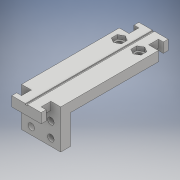
# Autodesk Inventor part: Attachment
Saved by Autodesk Inventor 2018 (Build 220112000, 112)
## iProperties
Created: 2018-05-09
Part Number: Attachment
Material: Generic
Document SubType Name: Modeling
Designer: s4321966
Density: 1 g/cm^3
Appearance: Default
Mass: 6.80777 g
Surface Area: 44.3396 cm^2
Volume: 6.80777 cm^3
Author: s4321966
Autodesk Inventor part; units mm, degrees
ref_plane "YZ Plane" through (0, 0, 0) normal (1, 0, 0) x (0, 1, 0)
ref_plane "XZ Plane" through (0, 0, 0) normal (0, 1, 0) x (-1, 0, 0)
ref_plane "XY Plane" through (0, 0, 0) normal (0, 0, 1) x (1, 0, 0)
sketch "Sketch1" plane through (0, 0, 0) normal (0, 0, 1) x (1, 0, 0)
  line L0 (0, 0) -> (20, 0)
  line L1 (20, 0) -> (20, -2.7984)
  line L2 (0, -2.7984) -> (0, 0)
  line L3 (0, 0) -> (20, 0)
  line L4 (20, 0) -> (20, -50)
  line L5 (20, -50) -> (0, -50)
  line L6 (0, -50) -> (0, 0)
  line L7 (0, 0) -> (5, 0)
  line L8 (0, -5) -> (0, 0)
  circle A0 centre (5, -5) radius 1.651
  line L9 (20, 0) -> (15, 0)
  line L10 (15, -5) -> (20, -5)
  line L11 (20, -5) -> (20, 0)
  circle A1 centre (15, -5) radius 1.651
  dimension "d1" = 20
  dimension "d2" = 50
  dimension "d6" = 5
  dimension "d7" = 5
  dimension "d9" = 3.302
  constraints: 24 end point, 4 horizontal, 4 parallel, 2 centre point, 2 perpendicular
  measures "d1" distance of L4.end L5.end
  measures "d2" distance of L3.end L4.end
  measures "d6" distance of L10.end L10.start
  measures "d7" distance of L10.start L9.end
  measures "d9" diameter of A1
extrude "Extrusion1" add sketch "Sketch1" along normal blind 5
sketch "Sketch2" plane through (0, 0, 5) normal (0, 0, 1) x (1, 0, 0)
  line L0 (20, 0) -> (0, 0) projected
  line L1 (10, 0) -> (5, 0)
  line L2 (5, 0) -> (5, 5)
  line L3 (5, 5) -> (10, 5)
  line L4 (10, 5) -> (10, 0)
  line L5 (10, 5) -> (2.5, 5)
  line L6 (2.5, 5) -> (2.5, 7.5)
  line L7 (2.5, 7.5) -> (10, 7.5)
  line L8 (10, 7.5) -> (10, 5)
  line L9 (2.5, 7.5) -> (17.5, 7.5)
  line L10 (17.5, 7.5) -> (17.5, 5)
  line L11 (17.5, 5) -> (2.5, 5)
  line L12 (2.5, 5) -> (2.5, 7.5)
  line L13 (10, 5) -> (15, 5)
  line L14 (15, 5) -> (15, 0)
  line L15 (15, 0) -> (10, 0)
  line L16 (10, 0) -> (10, 5)
  dimension "d12" = 5
  dimension "d13" = 5
  dimension "d14" = 7.5
  dimension "d15" = 2.5
  dimension "d16" = 15
  dimension "d17" = 2.5
  dimension "d18" = 5
  dimension "d19" = 5
  constraints: 32 end point, 8 parallel, 4 horizontal, 4 perpendicular, 1 midpoint
  measures "d12" distance of L2.end L3.end
  measures "d13" distance of L1.end L2.end
  measures "d14" distance of L6.end L7.end
  measures "d15" distance of L5.end L6.end
  measures "d16" distance of L10.end L11.end
  measures "d17" distance of L9.end L10.end
  measures "d18" distance of L14.end L15.end
  measures "d19" distance of L13.end L14.end
extrude "Extrusion2" add sketch "Sketch2" against normal blind 5
sketch "Sketch3" plane through (0, 0, 0) normal (0, 0, -1) x (-1, 0, 0)
  line L0 (-5, 0) -> (-5, 5) projected
  line L1 (-5, 0) -> (-15, 0)
  line L2 (-15, 0) -> (-15, 5)
  line L3 (-15, 5) -> (-5, 5)
  line L4 (-5, 5) -> (-5, 0)
  point P0 (0, 0)
  constraints: 8 end point, 2 parallel, 1 horizontal, 1 perpendicular
extrude "Extrusion3" cut sketch "Sketch3" against normal blind 1
sketch "Sketch4" plane through (0, 0, 0) normal (0, 0, -1) x (-1, 0, 0)
  line L0 (-5, 0) -> (0, 0) projected
  line L1 (-20, -50) -> (0, -50) projected
  line L2 (0, 0) -> (-20, 0)
  line L3 (-20, 0) -> (-20, -50)
  line L4 (-20, -50) -> (0, -50)
  line L5 (0, -50) -> (0, 0)
  line L6 (0, -50) -> (-5, -50)
  line L7 (-5, -50) -> (-5, -30)
  line L8 (-5, -30) -> (0, -30)
  line L9 (0, -30) -> (0, -50)
  line L10 (0, -50) -> (0, 0) projected
  line L11 (0, -50) -> (-5, -50)
  line L12 (-5, -50) -> (-5, -30)
  line L13 (-5, -30) -> (0, -30)
  line L14 (0, -30) -> (0, -50)
  line L15 (0, -50) -> (-20, -50)
  line L16 (-20, -50) -> (-20, -45)
  line L17 (-20, -45) -> (0, -45)
  line L18 (0, -45) -> (0, -50)
  dimension "d28" = 5
  dimension "d29" = 20
  dimension "d30" = 5
  dimension "d31" = 20
  dimension "d32" = 20
  dimension "d33" = 5
  constraints: 32 end point, 8 parallel, 4 horizontal, 4 perpendicular
  measures "d28" distance of L7.end L8.end
  measures "d29" distance of L6.end L7.end
  measures "d30" distance of L7.end L13.end
  measures "d31" distance of L11.end L7.end
  measures "d32" distance of L16.end L17.end
  measures "d33" distance of L15.end L16.end
extrude "Extrusion4" add sketch "Sketch4" along normal blind 15 contours L17 L7 L1 L3 | L5 L1 L7 L17
sketch "Sketch5" plane through (0, 0, 5) normal (0, 0, 1) x (1, 0, 0)
  line L0 (20, -50) -> (20, 0) projected
  line L1 (20, 0) -> (0, 0)
  line L2 (0, 0) -> (0, -50)
  line L3 (0, -50) -> (20, -50)
  line L4 (20, -50) -> (20, 0)
  line L5 (10, -50) -> (15, -50)
  line L6 (15, -50) -> (15, -55)
  line L7 (15, -55) -> (10, -55)
  line L8 (10, -55) -> (10, -50)
  line L9 (15, -55) -> (5, -55)
  line L10 (5, -55) -> (5, -50)
  line L11 (5, -50) -> (15, -50)
  line L12 (15, -50) -> (15, -55)
  line L13 (10, -55) -> (17.5, -55)
  line L14 (17.5, -55) -> (17.5, -57.5)
  line L15 (17.5, -57.5) -> (10, -57.5)
  line L16 (10, -57.5) -> (10, -55)
  line L17 (17.5, -57.5) -> (2.5, -57.5)
  line L18 (2.5, -57.5) -> (2.5, -55)
  line L19 (2.5, -55) -> (17.5, -55)
  line L20 (17.5, -55) -> (17.5, -57.5)
  dimension "d36" = 5
  dimension "d37" = 5
  dimension "d38" = 10
  dimension "d39" = 5
  dimension "d40" = 7.5
  dimension "d41" = 2.5
  dimension "d42" = 15
  dimension "d43" = 2.5
  constraints: 40 end point, 10 parallel, 5 horizontal, 5 perpendicular, 1 midpoint
  measures "d36" distance of L6.end L7.end
  measures "d37" distance of L5.end L6.end
  measures "d38" distance of L10.end L11.end
  measures "d39" distance of L9.end L10.end
  measures "d40" distance of L14.end L15.end
  measures "d41" distance of L13.end L14.end
  measures "d42" distance of L18.end L19.end
  measures "d43" distance of L17.end L18.end
extrude "Extrusion5" add sketch "Sketch5" against normal blind 5 contours L6 L7 L8 L3 | L8 L9 L10 L3 | L13 L14 L15 L16 L7 | L16 L17 L18 L19 L9
sketch "Sketch6" plane through (0, 0, 0) normal (0, 0, -1) x (-1, 0, 0)
  line L0 (-5, -55) -> (-5, -50) projected
  line L1 (-15, -50) -> (-5, -50) projected
  line L2 (-5, -55) -> (-15, -55)
  line L3 (-15, -55) -> (-15, -50)
  line L4 (-15, -50) -> (-5, -50)
  line L5 (-5, -50) -> (-5, -55)
  point P0 (0, 0)
  constraints: 8 end point, 2 parallel, 1 horizontal, 1 perpendicular
extrude "Extrusion6" cut sketch "Sketch6" against normal blind 1
sketch "Sketch8" plane through (0, -45, 0) normal (0, 1, 0) x (1, 0, 0)
  line L0 (0, 15) -> (20, 15) projected
  line L1 (0, 15) -> (20, 15)
  line L2 (20, 15) -> (20, 0)
  line L3 (20, 0) -> (0, 0)
  line L4 (0, 0) -> (0, 15)
  line L5 (0, 0) -> (0, 15) projected
  line L6 (0, 7.5) -> (20, 7.5)
  line L7 (20, 0) -> (20, 15) projected
  line L8 (20, 0) -> (0, 15)
  line L9 (20, 15) -> (0, 0)
  line L10 (10, 7.5) -> (10, 15)
  line L11 (10, 7.5) -> (10, 0)
  line L12 (10, 7.5) -> (0, 0)
  line L13 (10, 7.5) -> (20, 0)
  line L14 (10, 7.5) -> (0, 15)
  line L15 (10, 7.5) -> (20, 15)
  circle A0 centre (5, 3.75) radius 1.651
  circle A1 centre (15, 3.75) radius 1.651
  circle A2 centre (15, 11.25) radius 1.651
  circle A3 centre (5, 11.25) radius 1.651
  dimension "d48" = 3.302
  dimension "d49" = 3.302
  dimension "d50" = 3.302
  dimension "d51" = 3.302
  constraints: 26 end point, 9 midpoint, 4 centre point, 4 collinear, 2 parallel, 1 horizontal, 1 perpendicular
  measures "d48" diameter of A0
  measures "d49" diameter of A1
  measures "d50" diameter of A2
  measures "d51" diameter of A3
extrude "Extrusion7" cut sketch "Sketch8" against normal blind 5 contours A3 L8 | L8 A3 | A2 L9 | L9 A2 | A1 L8 | L8 A1 | A0 L9 | L9 A0
sketch "Sketch9" plane through (2.5, -57.5, 5) normal (0, -1, 0) x (1, 0, 0)
  line L0 (15, 0) -> (0, 0) projected
  line L1 (7.5, 0) -> (8, 0)
  line L2 (8, 0) -> (8, -0.5)
  line L3 (8, -0.5) -> (7.5, -0.5)
  line L4 (7.5, -0.5) -> (7.5, 0)
  line L5 (7.5, 0) -> (7, 0)
  line L6 (7, 0) -> (7, -0.5)
  line L7 (7, -0.5) -> (7.5, -0.5)
  line L8 (7.5, -0.5) -> (7.5, 0)
  point P0 (-2.5, -5)
  dimension "d54" = 0.5
  dimension "d55" = 0.5
  dimension "d56" = 0.5
  dimension "d57" = 0.5
  constraints: 16 end point, 4 parallel, 2 horizontal, 2 perpendicular, 1 midpoint
  measures "d54" distance of L2.end L3.end
  measures "d55" distance of L1.end L2.end
  measures "d56" distance of L7.end L6.end
  measures "d57" distance of L6.end L5.end
extrude "Extrusion8" cut sketch "Sketch9" against normal blind 500
sketch "Sketch10" plane through (0, -45, 0) normal (0, 1, 0) x (1, 0, 0)
  circle A0 centre (5, 11.25) radius 1.651 projected
  circle A1 centre (5, 11.25) radius 1.651
  circle A2 centre (5, 3.75) radius 1.651 projected
  circle A3 centre (5, 3.75) radius 1.651
  circle A4 centre (15, 11.25) radius 1.651 projected
  circle A5 centre (15, 11.25) radius 1.651
  circle A6 centre (15, 3.75) radius 1.651 projected
  circle A7 centre (15, 3.75) radius 1.651
  circle A8 centre (5, 11.25) radius 3
  circle A9 centre (15, 11.25) radius 3
  circle A10 centre (5, 3.75) radius 3
  circle A11 centre (15, 3.75) radius 3
  line L0 (5, 14.25) -> (7.5981, 12.75)
  line L1 (7.5981, 12.75) -> (7.5981, 9.75)
  line L2 (7.5981, 9.75) -> (5, 8.25)
  line L3 (5, 8.25) -> (2.4019, 9.75)
  line L4 (2.4019, 9.75) -> (2.4019, 12.75)
  line L5 (2.4019, 12.75) -> (5, 14.25)
  line L6 (15, 14.25) -> (17.5981, 12.75)
  line L7 (17.5981, 12.75) -> (17.5981, 9.75)
  line L8 (17.5981, 9.75) -> (15, 8.25)
  line L9 (15, 8.25) -> (12.4019, 9.75)
  line L10 (12.4019, 9.75) -> (12.4019, 12.75)
  line L11 (12.4019, 12.75) -> (15, 14.25)
  line L12 (5, 6.75) -> (7.5981, 5.25)
  line L13 (7.5981, 5.25) -> (7.5981, 2.25)
  line L14 (7.5981, 2.25) -> (5, 0.75)
  line L15 (5, 0.75) -> (2.4019, 2.25)
  line L16 (2.4019, 2.25) -> (2.4019, 5.25)
  line L17 (2.4019, 5.25) -> (5, 6.75)
  line L18 (15, 6.75) -> (17.5981, 5.25)
  line L19 (17.5981, 5.25) -> (17.5981, 2.25)
  line L20 (17.5981, 2.25) -> (15, 0.75)
  line L21 (15, 0.75) -> (12.4019, 2.25)
  line L22 (12.4019, 2.25) -> (12.4019, 5.25)
  line L23 (12.4019, 5.25) -> (15, 6.75)
  point P0 (0, 0)
  dimension "d60" = 6
  dimension "d61" = 6
  dimension "d62" = 6
  dimension "d63" = 6
  constraints: 48 end point, 12 coincident, 4 centre point, 4 vertical alignment, 60 other
extrude "Extrusion9" cut sketch "Sketch10" against normal blind 2 contours L1 L2 L3 L4 L5 L0 | L7 L8 L9 L10 L11 L6 | L13 L14 L15 L16 L17 L12 | L19 L20 L21 L22 L23 L18
sketch "Sketch11" plane through (0, 0, 5) normal (0, 0, 1) x (1, 0, 0)
  circle A0 centre (5, -5) radius 1.651 projected
  circle A1 centre (5, -5) radius 3
  circle A2 centre (15, -5) radius 1.651 projected
  circle A3 centre (15, -5) radius 3
  line L0 (5, -2) -> (7.5981, -3.5)
  line L1 (7.5981, -3.5) -> (7.5981, -6.5)
  line L2 (7.5981, -6.5) -> (5, -8)
  line L3 (5, -8) -> (2.4019, -6.5)
  line L4 (2.4019, -6.5) -> (2.4019, -3.5)
  line L5 (2.4019, -3.5) -> (5, -2)
  line L6 (15, -2) -> (17.5981, -3.5)
  line L7 (17.5981, -3.5) -> (17.5981, -6.5)
  line L8 (17.5981, -6.5) -> (15, -8)
  line L9 (15, -8) -> (12.4019, -6.5)
  line L10 (12.4019, -6.5) -> (12.4019, -3.5)
  line L11 (12.4019, -3.5) -> (15, -2)
  point P0 (0, 0)
  dimension "d66" = 6
  dimension "d67" = 6
  constraints: 24 end point, 4 coincident, 2 vertical alignment, 30 other
extrude "Extrusion10" cut sketch "Sketch11" against normal blind 2 contours L1 L2 L3 L4 L5 L0 | L7 L8 L9 L10 L11 L6
body "Solid1"
